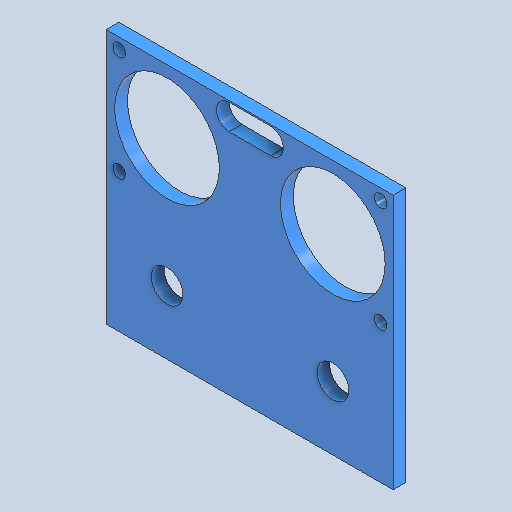
# Autodesk Inventor part: suporte_ultrassonico_001
Saved by Autodesk Inventor 2026 (Build 300175000, 175)
## iProperties
Created: 2025-05-28
Part Number: suporte_ultrassonico_001
Material: ABS Plastic
Document SubType Name: Modeling
Designer: Carlos Dias
Density: 1.06 g/cm^3
Appearance: Smooth - White
Finish1_Area: 1627,116 mm^2
Finish1_Appearance: Cyan
Finish2_Area: 3284,550 mm^2
Finish2_Appearance: Cyan
Author: Carlos Dias
## iProperties of the stored document suporte_ultrassonico_001_3DPrint.ipt
Created: 2025-05-29
Part Number: suporte_ultrassonico_001_3DPrint
Material: Generic
Document SubType Name: Modeling
Designer: Carlos Dias
Density: 1 g/cm^3
Appearance: Default
Author: Carlos Dias
Autodesk Inventor part; units mm, degrees
sketch "Sketch1" plane through (0, 0, 0) normal (0, 0, 1) x (1, 0, 0)
  line L0 (-22.5, 20) -> (22.5, 20)
  line L1 (22.5, 20) -> (22.5, 0)
  line L2 (22.5, 0) -> (-22.5, 0)
  line L3 (-22.5, 0) -> (-22.5, 20)
  line L4 (-22.5, 20) -> (22.5, 0) construction
  line L5 (22.5, 20) -> (-22.5, 0) construction
  circle A0 centre (-20.4468, 18.2798) radius 1
  circle A1 centre (20.5532, 18.2798) radius 1
  circle A2 centre (20.5532, 1.7798) radius 1
  circle A3 centre (-20.4468, 1.7798) radius 1
  circle A4 centre (-12.9468, 10.0298) radius 8.2
  circle A5 centre (13.0532, 10.0298) radius 8.2
  line L6 (-3.1968, 19.7798) -> (3.3032, 19.7798)
  line L7 (-3.1968, 15.7798) -> (3.3032, 15.7798)
  arc A6 (-3.1968, 19.7798) -> (-3.1968, 15.7798) centre (-3.1968, 17.7798) ccw
  arc A7 (3.3032, 15.7798) -> (3.3032, 19.7798) centre (3.3032, 17.7798) ccw
  line L8 (-22.5, 0) -> (22.5, 0)
  line L9 (22.5, 0) -> (22.5, -20)
  line L10 (22.5, -20) -> (-22.5, -20)
  line L11 (-22.5, -20) -> (-22.5, 0)
  line L12 (-22.5, 0) -> (22.5, -20) construction
  line L13 (22.5, 0) -> (-22.5, -20) construction
  circle A8 centre (13.0532, -10) radius 2.5
  circle A9 centre (-12.9468, -10) radius 2.5
  circle A10 centre (-20.4468, 18.2798) radius 1 projected
  circle A11 centre (-20.4468, 1.7798) radius 1 projected
  circle A12 centre (20.5532, 18.2798) radius 1 projected
  circle A13 centre (20.5532, 1.7798) radius 1 projected
  point P0 (0, 0)
  point P1 (0, 10)
  point P2 (-5.1968, 17.7798)
  point P3 (0, 0)
  point P4 (5.3032, 17.7798)
  point P5 (0, -10)
  point P6 (-22.5, 0)
  dimension "d0" = 45
  dimension "d1" = 20
  dimension "d16" = 16.4
  dimension "d18" = 12.9468
  dimension "d19" = 9.9702
  dimension "d20" = 9.9702
  dimension "d21" = 13.0532
  dimension "d23" = 10.5
  dimension "d24" = 2
  dimension "d25" = 5
  dimension "d26" = 20
  constraints: 28 end point, 10 centre point, 9 equal radius, 6 point on circle, 5 midpoint, 5 vertical alignment, 4 coincident, 4 horizontal, 4 horizontal alignment, 4 parallel, 2 perpendicular
  measures "d0" distance of L0.start L0.end
  measures "d1" distance of L0.end L1.end
  measures "d16" diameter of A4
  measures "d18" horizontal distance of point (0, 0) A4.centre
  measures "d19" distance from line of L0 A4.centre
  measures "d20" distance from line of L0 A5.centre
  measures "d21" horizontal distance of point (0, 0) A5.centre
  measures "d23" distance of point (-5.197, 17.78) point (5.303, 17.78)
  measures "d24" radius of A6
  measures "d25" diameter of A8
  measures "d26" distance between parallel lines of L10 L2
extrude "Extrusion2" add sketch "Sketch1" along normal mid plane 2
body "Solid2"
